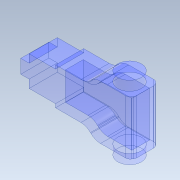
# Autodesk Inventor part: body_2
Saved by Autodesk Inventor 2020 (Build 240168000, 168)
## iProperties
Created: 2021-03-27
Part Number: body_2
Material: Generic
Document SubType Name: Modeling
Designer: DELL
Density: 1 g/cm^3
Appearance: Clear - Blue
Author: DELL
Autodesk Inventor part; units mm, degrees
ref_plane "YZ Plane" through (0, 0, 0) normal (1, 0, 0) x (0, 1, 0)
ref_plane "XZ Plane" through (0, 0, 0) normal (0, 1, 0) x (-1, 0, 0)
ref_plane "XY Plane" through (0, 0, 0) normal (0, 0, 1) x (1, 0, 0)
sketch "Sketch1" plane through (0, 0, 0) normal (0, 0, 1) x (1, 0, 0)
  line L0 (-122, 0) -> (122, 0) construction
  line L1 (-122, 62) -> (-122, -62)
  circle A0 centre (-69.5, 54.5) radius 2.25
  line L2 (122, -70) -> (122, 70) construction
  line L3 (-114, 0) -> (-114, 54.5) construction
  line L4 (-114, 0) -> (-114, -54.5) construction
  circle A1 centre (-114.5, 54.5) radius 2.25
  circle A2 centre (-114.5, 54.5) radius 1.25
  circle A3 centre (-69.5, 54.5) radius 1.25
  line L5 (-122, 62) -> (-26.6066, 62)
  line L6 (-26.6066, 62) -> (1.3934, 90)
  line L7 (1.3934, 90) -> (122, 90)
  line L8 (122, 90) -> (122, 0)
  line L9 (122, -90) -> (122, 0)
  line L10 (1.3934, -90) -> (122, -90)
  line L11 (-26.6066, -62) -> (1.3934, -90)
  line L12 (-122, -62) -> (-26.6066, -62)
  line L13 (107, 75) -> (7.6066, 75)
  line L14 (7.6066, 75) -> (-20.3934, 47)
  line L15 (-20.3934, 47) -> (-114, 47)
  line L16 (-114, -47) -> (-20.3934, -47)
  line L17 (-20.3934, -47) -> (7.6066, -75)
  line L18 (7.6066, -75) -> (107, -75)
  line L19 (114.5, 82.5) -> (4.5, 82.5) construction
  line L20 (4.5, 82.5) -> (-23.5, 54.5) construction
  line L21 (-23.5, 54.5) -> (-114.5, 54.5) construction
  line L22 (-114.5, 54.5) -> (-114.5, -54.5) construction
  line L23 (-114.5, -54.5) -> (-23.5, -54.5) construction
  line L24 (-23.5, -54.5) -> (4.5, -82.5) construction
  line L25 (4.5, -82.5) -> (114.5, -82.5) construction
  line L26 (114.5, -82.5) -> (114.5, 0) construction
  line L27 (114.5, 0) -> (114.5, 82.5) construction
  line L28 (107, 75) -> (107, -75)
  line L29 (-122, 62) -> (-130, 62)
  line L30 (-130, 62) -> (-130, -62)
  line L31 (-130, -62) -> (-122, -62)
  line L32 (-122, -62) -> (-122, 62)
  line L33 (122, 0) -> (-130, 0)
  circle A4 centre (42, 82.5) radius 1.25
  circle A5 centre (42, 82.5) radius 2.25
  circle A6 centre (102, 82.5) radius 1.25
  circle A7 centre (102, 82.5) radius 2.25
  line L34 (72, 90) -> (72, 75) construction
  circle A8 centre (-9.5, 68.5) radius 1.25
  circle A9 centre (-9.5, 68.5) radius 2.25
  line L35 (-114, 47) -> (-114, -47)
  circle A10 centre (-118, 0) radius 2.25
  circle A11 centre (-118, 0) radius 1.25
  circle A12 centre (-126, 30) radius 2.25
  circle A13 centre (-126, 30) radius 1.25
  circle A14 centre (-126, -30) radius 2.25
  circle A15 centre (-126, -30) radius 1.25
  line L36 (-126, 62) -> (-126, -62) construction
  point P0 (0, 0)
  point P1 (0, 0)
  point P2 (0, 0)
  point P3 (0, 0)
  dimension "d0" = 124
  dimension "d1" = 8
  dimension "d2" = 244
  dimension "d15" = 15
  dimension "d16" = 122
  dimension "d17" = 7.5
  dimension "d18" = 4.5
  dimension "d19" = 2.5
  dimension "d20" = 45
  dimension "d21" = 180
  dimension "d22" = 15
  dimension "d24" = 8
  dimension "d28" = 20
  dimension "d29" = 50
  dimension "d30" = 60
  dimension "d31" = 28
  dimension "d40" = 30
  dimension "d41" = 4
  constraints: 74 end point, 16 centre point, 14 equal radius, 12 point on line, 11 coincident, 8 midpoint, 6 parallel, 6 symmetric about line, 3 collinear, 2 horizontal, 2 perpendicular, 1 vertical, 16 other
  measures "d0" distance of L29.start L12.start
  measures "d1" distance between parallel lines of L1 L3
  measures "d2" distance between parallel lines of L1 L2
  measures "d15" distance between parallel lines of L7 L13
  measures "d16" distance from line of point (0, 0) L1
  measures "d17" distance between parallel lines of L7 L19
  measures "d18" diameter of A1
  measures "d19" diameter of A2
  measures "d20" distance of A1.centre A3.centre
  measures "d21" distance between parallel lines of L10 L7
  measures "d22" distance between parallel lines of L9 L28
  measures "d24" distance between parallel lines of L1 L30
  measures "d28" distance from line of L8 A6.centre
  measures "d29" distance between parallel lines of L8 L34
  measures "d30" horizontal distance of A3.centre A8.centre
  measures "d31" horizontal distance of L6.start L6.end
  measures "d40" distance from line of L33 A12.centre
  measures "d41" distance from line of L1 A10.centre
extrude "Extrusion1" add sketch "Sketch1" along normal mid plane 94 contours L5 L6 L7 L8 L33 L28 L13 L14 L15 L35 A10 L1 | L1 L33 L30 L29 | L33 A10 L35 L16 L17 L18 L28 L9 L10 L11 L12 L1 | L1 L31 L30 L33 | A10 L33 A11 | L33 A11 A10 | A11 L33 | L33 A11 | L35 L15 L14 L13 L28 L33 | L33 L28 L18 L17 L16 L35 | A0 | A1 | A2 | A3 | A4 | A5 | A6 | A7 | A8 | A9 | A12 | A13 | A14 | A15
extrude "Extrusion2" cut sketch "Sketch1" along normal mid plane 59 contours L35 L15 L14 L13 L28 L33 | L33 L28 L18 L17 L16 L35
sketch "Sketch2" plane through (-130, -62, 47) normal (-1, 0, 0) x (0, 0, 1)
  line L0 (0, -28) -> (0, 152) projected
  line L1 (-94, 12) -> (0, 12)
  line L2 (0, 12) -> (0, 112)
  line L3 (0, 112) -> (-94, 112)
  line L4 (-94, 112) -> (-94, 12)
  line L5 (-94, 12) -> (0, 112) construction
  line L6 (0, 12) -> (-94, 112) construction
  line L7 (-94, 39) -> (0, 39)
  line L8 (0, 39) -> (0, 85)
  line L9 (0, 85) -> (-94, 85)
  line L10 (-94, 85) -> (-94, 39)
  line L11 (-94, 39) -> (0, 85) construction
  line L12 (0, 39) -> (-94, 85) construction
  point P0 (-47, 62)
  dimension "d52" = 100
  dimension "d55" = 46
  constraints: 24 end point, 4 midpoint, 4 parallel, 2 horizontal, 2 perpendicular, 2 point on line
  measures "d52" distance between parallel lines of L1 L3
  measures "d55" distance between parallel lines of L7 L9
extrude "Extrusion3" add sketch "Sketch2" along normal blind 88
extrude "Extrusion4" add sketch "Sketch2" along normal blind 116 contours L7 L4 L9 L0
sketch "Sketch3" plane through (0, 0, 0) normal (0, 1, 0) x (-1, 0, 0)
  circle A0 centre (175, 0) radius 32
  line L0 (130, -47) -> (130, 47) projected
  line L1 (130, -47) -> (130, 47) projected
  line L2 (130, -47) -> (130, 47) construction
  line L3 (130, 0) -> (245.8238, 0) construction
  circle A1 centre (175, 0) radius 40
  line L4 (205.5437, 9.5437) -> (218, 22)
  line L5 (218, 22) -> (218, -22)
  line L6 (218, -22) -> (205.5437, -9.5437)
  line L7 (218, 47) -> (218, -47) projected
  line L8 (218, 47) -> (246, 47) projected
  line L9 (226, 47) -> (246, 20)
  line L10 (246, 20) -> (246, 47)
  line L11 (246, 47) -> (226, 47)
  line L12 (218, -47) -> (246, -47)
  line L13 (226, -47) -> (246, -20)
  line L14 (246, -20) -> (246, -47)
  line L15 (-122, 47) -> (-1.3934, 47) projected
  line L16 (-122, 47) -> (-122, 32)
  line L17 (-122, 32) -> (-112, 47)
  line L18 (-122, -47) -> (-1.3934, -47)
  line L19 (-122, -47) -> (-122, -32)
  line L20 (-122, -32) -> (-112, -47)
  circle A2 centre (-70, 0) radius 39.5
  line L21 (-122, -47) -> (-122, 47) projected
  point P0 (0, 0)
  point P1 (211.7631, 15.7631)
  point P2 (211.7631, -15.7631)
  dimension "d58" = 45
  dimension "d59" = 64
  dimension "d62" = 80
  dimension "d64" = 44
  dimension "d69" = 20
  dimension "d70" = 27
  dimension "d80" = 15
  dimension "d81" = 10
  dimension "d87" = 52
  dimension "d88" = 79
  constraints: 30 end point, 7 symmetric about line, 6 point on line, 3 centre point, 2 collinear, 2 perpendicular, 2 point on circle, 2 vertical, 1 coincident, 1 horizontal, 1 midpoint, 1 other
  measures "d58" distance from line of L0 A0.centre
  measures "d59" diameter of A0
  measures "d62" diameter of A1
  measures "d64" distance of L4.end L5.end
  measures "d69" horizontal distance of L9.start L9.end
  measures "d70" vertical distance of L9.start L9.end
  measures "d80" distance of L15.start L16.end
  measures "d81" horizontal distance of L16.end L17.end
  measures "d87" distance from line of L21 A2.centre
  measures "d88" diameter of A2
extrude "Extrusion9" cut sketch "Sketch3" against normal through all both and the other way through all contours L15 L17 L16 | L19 L20 L18
fillet "Fillet8" radius 45 8 edges at (1.3934, -90, 0) (-26.6066, -62, 0) (-20.3934, -47, 0) (7.6066, -75, 0) (-26.6066, 62, 0) (1.3934, 90, 0) (-20.3934, 47, 0) (7.6066, 75, 0)
fillet "Fillet9" radius 15 4 edges at (112, 0, 47) (122, 0, 32) (122, 0, -32) (112, 0, -47)
extrude "Extrusion14" add sketch "Sketch3" against normal blind 32 from surface at -90 contours A2
mirror "Mirror2" about plane through (0, 0, 0) normal (0, 1, 0) of "Extrusion14"
equation "\"d0\" = d45"
equation "\"d17\" = 0.5 * d15"
equation "\"d21\" = d47"
equation "\"d45\" = 124"
equation "\"d46\" = 12"
equation "\"d47\" = 180"
body "Solid1"
